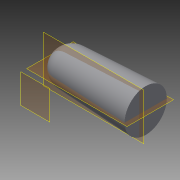
# Autodesk Inventor part: Muffler
Saved by Autodesk Inventor 2015 (Build 190159000, 159)
## iProperties
Created: 2016-02-28
Part Number: Muffler
Material: Generic
Document SubType Name: Modeling
Designer: Owner
Density: 1 g/cm^3
Appearance: Default
Author: Owner
Autodesk Inventor part; units mm, degrees
ref_plane "YZ Plane" through (0, 0, 0) normal (1, 0, 0) x (0, 1, 0)
ref_plane "Work Plane1" through (0, 0, 25.4) normal (0, 0, 1) x (1, 0, 0)
sketch "Sketch5" plane through (0, 0, 0) normal (0, 1, 0) x (-1, 0, 0)
  arc A0 (5.151, -16.51) -> (16.653, -4.445) centre (4.5714, -4.4424) ccw
  line L0 (16.653, -4.445) -> (-46.0487, -4.445)
  line L1 (-46.0487, -4.445) -> (-46.0487, -18.9693)
  line L2 (-30.48, -15.24) -> (0, -15.24)
  line L3 (-46.0487, -18.9693) -> (5.151, -16.51)
  point P0 (0, 0)
  point P1 (0, 0)
  point P2 (0, -12.065)
  dimension "d5" = 2.75
  dimension "d6" = 1.27
  dimension "d7" = 7.62
  constraints: 6 end point, 2 point on circle, 1 centre point, 1 perpendicular, 1 tangent, 1 vertical
  measures "d5" angle of L2 L3
  measures "d6" distance from line of L2 L3.end
  measures "d7" distance from line of L0 point (0, -12.065)
revolve "Revolution1" add sketch "Sketch5" angle 360 about axis through (-16.653, 0, -4.445) along (1, 0, 0)
body "Solid1"
